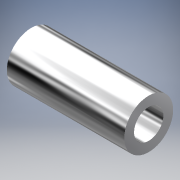
# Autodesk Inventor part: Spacer 24mm
Saved by Autodesk Inventor 2019.4 (Build 234330000, 330)
## iProperties
Created: 2020-01-01
Part Number: Spacer 24mm
Material: Aluminum 6061
Document SubType Name: Modeling
Designer: Mark
Mass: 3.2572 g
Surface Area: 13.069 cm^2
Volume: 1.20637 cm^3
Density: 2.7 g/cm^3
Appearance: Aluminum - Flat
Author: Mark
Autodesk Inventor part; units mm, degrees
ref_plane "YZ Plane" through (0, 0, 0) normal (1, 0, 0) x (0, 1, 0)
ref_plane "XZ Plane" through (0, 0, 0) normal (0, 1, 0) x (-1, 0, 0)
ref_plane "XY Plane" through (0, 0, 0) normal (0, 0, 1) x (1, 0, 0)
sketch "Sketch1" plane through (0, 0, 0) normal (1, 0, 0) x (0, 1, 0)
  circle A0 centre (58.1338, 0) radius 5
  circle A1 centre (58.1338, 0) radius 3
  point P0 (0, 0)
  dimension "d0" = 10
  dimension "d1" = 6
  constraints: 2 centre point, 1 coincident
  measures "d0" diameter of A0
  measures "d1" diameter of A1
extrude "Extrusion1" add sketch "Sketch1" along normal blind 24
body "Solid1"
